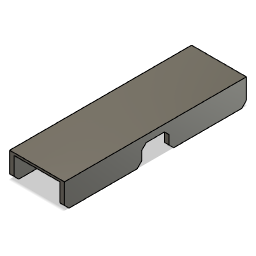
Sensor Bracket Top (Autodesk Fusion 360 design; units mm, degrees)
Autodesk Fusion 360 part; units mm, degrees
note: some values were not read from the file. Set by a fixed rule: which sketch regions a step uses.
sketch "Sketch1" plane through (0, 0, 0) normal (0, 0, 1) x (1, 0, 0)
  line L0 (10.05, -4.5) -> (-10.05, -4.5)
  line L1 (-10.05, -4.5) -> (-10.05, 4.5)
  line L2 (-10.05, 4.5) -> (10.05, 4.5)
  line L3 (10.05, 4.5) -> (10.05, -4.5)
  line L4 (10.05, -4.5) -> (-10.05, 4.5) construction
  line L5 (-10.05, -4.5) -> (10.05, 4.5) construction
  line L6 (12.05, -6.5) -> (-12.05, -6.5)
  line L7 (-12.05, -6.5) -> (-12.05, 6.5)
  line L8 (-12.05, 6.5) -> (12.05, 6.5)
  line L9 (12.05, 6.5) -> (12.05, -6.5)
  line L10 (-10.05, -4.5) -> (-12.05, -4.5)
  line L11 (10.05, -4.5) -> (12.05, -4.5)
  dimension "d1" = -2
  dimension "d2" = 20.1
  dimension "d3" = 9
  constraint horizontal L0
  constraint perpendicular L0 L1
  constraint parallel L0 L2
  constraint parallel L1 L3
  constraint coincident L4 origin
  constraint coincident L5 origin
  constraint coincident L7 L10.end
  constraint perpendicular L7 L10
  constraint coincident L9 L11.end
  constraint perpendicular L9 L11
  measures "d2" distance of L0.start L0.end
  measures "d3" distance of L0.start L2.end
extrude "Extrude1" add sketch "Sketch1" along normal mid plane 80 contours L1 L2 L3 L7 L8 L9 L10 L11
sketch "Sketch2" plane through (0, 0, 0) normal (1, 0, 0) x (0, 0, -1)
  line L0 (6, -4.5) -> (-6, -4.5)
  line L1 (-6, -4.5) -> (-6, 3.5)
  line L2 (-6, 3.5) -> (6, 3.5)
  line L3 (6, 3.5) -> (6, -4.5)
  line L4 (6, -4.5) -> (-6, 3.5) construction
  line L5 (-6, -4.5) -> (6, 3.5) construction
  line L6 (40, -4.5) -> (-40, -4.5)
  point P0 (0, -0.5)
  dimension "d6" = 12
  dimension "d7" = 8
  constraint horizontal L0
  constraint perpendicular L0 L1
  constraint parallel L0 L2
  constraint parallel L1 L3
  constraint coincident L4 P0
  constraint coincident L5 P0
  constraint coincident L0.start L6
  constraint vertical origin P0
  measures "d6" distance of L1.end L2.end
  measures "d7" distance of L0.start L2.end
extrude "Extrude2" cut sketch "Sketch2" along normal through all and the other way through all
chamfer "Chamfer1" distance 2 angle 45 8 edges at (11.05, -4.5, 6) (11.05, -4.5, -6) (-11.05, -4.5, 6) (-11.05, -4.5, -6) (11.05, -4.5, 40) (-11.05, -4.5, 40) (11.05, -4.5, -40) (-11.05, -4.5, -40)
chamfer "Chamfer2" distance 1 angle 45 2 edges at (0, 4.5, 40) (0, 4.5, -40)
chamfer "Chamfer3" distance 2 angle 45 4 edges at (-11.05, 3.5, 6) (-11.05, 3.5, -6) (11.05, 3.5, 6) (11.05, 3.5, -6)
sketch "Sketch3" plane through (0, 0, 0) normal (1, 0, 0) x (0, 0, -1)
  line L0 (39, 4.5) -> (-39, 4.5)
  line L1 (-39, 4.5) -> (39, 4.5)
  circle A0 centre (0, 4.5) radius 0.75
  circle A1 centre (-32, 4.5) radius 0.75
  circle A2 centre (-24, 4.5) radius 0.75
  circle A3 centre (-16, 4.5) radius 0.75
  circle A4 centre (-8, 4.5) radius 0.75
  circle A5 centre (8, 4.5) radius 0.75
  circle A6 centre (16, 4.5) radius 0.75
  circle A7 centre (24, 4.5) radius 0.75
  circle A8 centre (32, 4.5) radius 0.75
  dimension "d12" = 1.5
  dimension "d15" = 8
  dimension "d16" = 0
  constraint midpoint L0 A0.centre
  measures "d12" diameter of A0
extrude "Extrude3" add sketch "Sketch3" along normal up to surface (10.05 mm away) and the other way up to surface (10.05 mm away) contours L0 L1 A8 | L0 L1 A7 | L0 L1 A6 | L0 L1 A5 | L0 L1 A0 | L0 L1 A4 | L0 L1 A3 | L0 L1 A2 | L0 L1 A1 picked at (32.0159, 4.2134) picked at (23.8056, 4.2563) picked at (15.875, 4.0018) picked at (8.2472, 4.2458) picked at (0.2698, 4.0143) picked at (-7.7844, 4.1154) picked at (-16.1861, 4.2927) picked at (-24.1944, 4.2563) picked at (-32.1559, 4.23)
